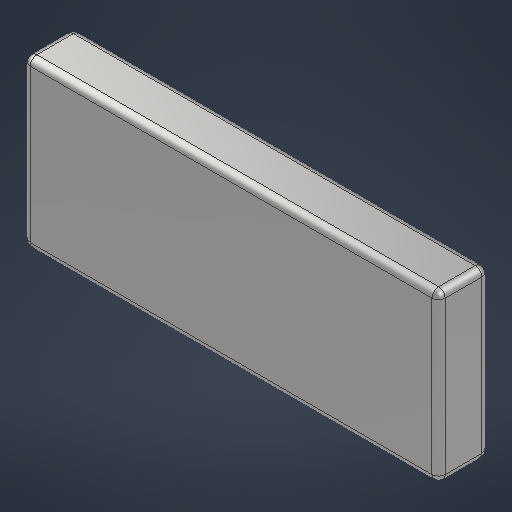
# Autodesk Inventor part: iman
Saved by Autodesk Inventor 2025 (Build 290162010, 162A)
## iProperties
Created: 2024-11-09
Part Number: iman
Material: Generic
Document SubType Name: Modeling
Designer: river
Density: 1 g/cm^3
Appearance: Default
Author: river
Autodesk Inventor part; units mm, degrees
ref_plane "YZ Plane" through (0, 0, 0) normal (1, 0, 0) x (0, 1, 0)
ref_plane "XZ Plane" through (0, 0, 0) normal (0, 1, 0) x (-1, 0, 0)
ref_plane "XY Plane" through (0, 0, 0) normal (0, 0, 1) x (1, 0, 0)
sketch "Sketch1" plane through (0, 0, 0) normal (0, 1, 0) x (-1, 0, 0)
  line L0 (-12.5, -1.5) -> (12.5, -1.5)
  line L1 (12.5, -1.5) -> (12.5, 1.5)
  line L2 (12.5, 1.5) -> (-12.5, 1.5)
  line L3 (-12.5, 1.5) -> (-12.5, -1.5)
  line L4 (-12.5, -1.5) -> (12.5, 1.5) construction
  line L5 (12.5, -1.5) -> (-12.5, 1.5) construction
  point P0 (0, 0)
  dimension "d0" = 25
  dimension "d1" = 3
  constraints: 12 end point, 2 midpoint, 2 parallel, 1 horizontal, 1 perpendicular
  measures "d0" distance of L2.end L1.end
  measures "d1" distance of L1.end L0.end
extrude "Extrusion1" add sketch "Sketch1" along normal blind 10
fillet "Fillet1" radius 0.4 12 edges at (0, 10, 1.5) (-12.5, 10, 0) (-12.5, 5, 1.5) (0, 10, -1.5) (12.5, 10, 0) (12.5, 5, 1.5) (12.5, 5, -1.5) (12.5, 0, 0) (0, 0, 1.5) (0, 0, -1.5) (-12.5, 5, -1.5) (-12.5, 0, 0)
body "Solid1"
